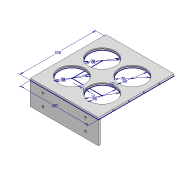
# Autodesk Inventor part: LensHolder
Saved by Autodesk Inventor 2020.3 (Build 243373010, 373A)
## iProperties
Created: 2020-12-03
Part Number: LensHolder
Material: Generic
Document SubType Name: Modeling
Designer: Yusuf
Mass: 169.587 g
Surface Area: 740.889 cm^2
Volume: 169.587 cm^3
Density: 1 g/cm^3
Appearance: Default
Author: Yusuf
Autodesk Inventor part; units mm, degrees
ref_plane "YZ Plane" through (0, 0, 0) normal (1, 0, 0) x (0, 1, 0)
ref_plane "XZ Plane" through (0, 0, 0) normal (0, 1, 0) x (-1, 0, 0)
ref_plane "XY Plane" through (0, 0, 0) normal (0, 0, 1) x (1, 0, 0)
sketch "Sketch1" plane through (0, 0, 0) normal (0, 1, 0) x (-1, 0, 0)
  line L0 (0, 0) -> (180, 0)
  line L1 (180, 0) -> (180, 200)
  line L2 (180, 200) -> (0, 200)
  line L3 (0, 200) -> (0, 0)
  circle A0 centre (130, 140) radius 35
  circle A1 centre (130, 60) radius 35
  circle A2 centre (50, 140) radius 35
  circle A3 centre (50, 60) radius 35
  line L4 (130, 140) -> (50, 140)
  line L5 (130, 140) -> (130, 60)
  circle A4 centre (130, 140) radius 34
  circle A5 centre (130, 60) radius 34
  circle A6 centre (50, 140) radius 34
  circle A7 centre (50, 60) radius 34
  point P0 (90, 140)
  point P1 (90, 200)
  point P2 (130, 100)
  point P3 (180, 100)
  dimension "d0" = 180
  dimension "d1" = 200
  dimension "d2" = 70
  dimension "d3" = 70
  dimension "d4" = 70
  dimension "d5" = 70
  dimension "d6" = 10
  dimension "d7" = 10
  dimension "d11" = 68
  dimension "d12" = 68
  dimension "d13" = 68
  dimension "d14" = 68
  constraints: 12 end point, 8 centre point, 4 coincident, 4 midpoint, 3 horizontal alignment, 3 vertical alignment, 2 horizontal, 2 parallel, 1 perpendicular, 1 vertical
  measures "d0" distance of L2.end L1.end
  measures "d1" distance of L1.end L0.end
  measures "d2" diameter of A0
  measures "d3" diameter of A1
  measures "d4" diameter of A2
  measures "d5" diameter of A3
  measures "d11" diameter of A4
  measures "d12" diameter of A5
  measures "d13" diameter of A6
  measures "d14" diameter of A7
extrude "Extrusion1" add sketch "Sketch1" along normal blind 5 contours L3 L2 L1 L0
extrude "Extrusion2" add sketch "Sketch1" along normal blind 3 contours A0 L5 A4 L4 | L4 A4 L5 A0 | A1 | A2 | A3
sketch "Sketch2" plane through (0, 0, 200) normal (1, 0, 0) x (0, 0, -1)
  circle A0 centre (40, 2.5) radius 1
  circle A1 centre (80, 2.5) radius 1
  circle A2 centre (120, 2.5) radius 1
  circle A3 centre (160, 2.5) radius 1
  line L0 (0, 0) -> (0, 5) projected
  line L1 (200, 0) -> (200, 5) projected
  line L2 (0, 5) -> (200, 5) projected
  dimension "d18" = 2
  dimension "d19" = 2
  dimension "d20" = 2
  dimension "d21" = 2
  dimension "d23" = 40
  dimension "d24" = 40
  dimension "d25" = 40
  dimension "d26" = 40
  dimension "d45" = 2.5
  constraints: 4 centre point, 3 horizontal alignment
  measures "d18" diameter of A0
  measures "d19" diameter of A1
  measures "d20" diameter of A2
  measures "d21" diameter of A3
  measures "d23" distance from line of L1 A3.centre
  measures "d24" distance of A3.centre A2.centre
  measures "d25" distance of A1.centre A2.centre
  measures "d26" distance of A1.centre A0.centre
  measures "d45" distance from line of L2 A1.centre
hole "Hole1" at (0, 2.5, 40) at (0, 2.5, 80) at (0, 2.5, 120) at (0, 2.5, 160) direction (-1, 0, 0) diameter 3.242 depth 11.8 thread size "M4x0.7" class "6H" standard "ANSI Metric M Profile"
sketch "Sketch3" plane through (0, 0, 0) normal (0, -1, 0) x (1, 0, 0)
  line L0 (0, 200) -> (0, 0) projected
  line L1 (-180, 0) -> (-180, 200) projected
  line L2 (0, 200) -> (-180, 200)
  line L3 (-180, 200) -> (-180, 194)
  line L4 (-180, 194) -> (0, 194)
  line L5 (0, 194) -> (0, 200)
  dimension "d35" = 6
  constraints: 8 end point, 2 parallel, 1 horizontal, 1 perpendicular, 1 point on line
  measures "d35" distance of L3.end L2.end
extrude "Extrusion3" add sketch "Sketch3" along normal blind 60
sketch "Sketch4" plane through (0, 0, 194) normal (0, 0, -1) x (-1, 0, 0)
  circle A0 centre (33.7554, -11.723) radius 5.5293
  circle A1 centre (33.7554, -43.277) radius 5.535
  circle A2 centre (146.2446, -11.723) radius 5.926
  circle A3 centre (146.2446, -43.277) radius 6.0534
  line L0 (33.7554, -11.723) -> (33.7554, -43.277)
  line L1 (33.7554, -11.723) -> (146.2446, -11.723)
  line L2 (0, 0) -> (180, 0) projected
  line L3 (0, -60) -> (0, 5) projected
  point P0 (90, -11.723)
  point P1 (90, 0)
  point P2 (33.7554, -27.5)
  point P3 (0, -27.5)
  constraints: 4 centre point, 4 end point, 4 midpoint, 3 horizontal alignment, 3 vertical alignment
hole "Hole2" at (-33.7554, -11.723, 194) at (-33.7554, -43.277, 194) at (-146.2446, -11.723, 194) at (-146.2446, -43.277, 194) direction (0, 0, 1) diameter 4.917 depth 17.1 thread size "M6x1" class "6H" standard "ANSI Metric M Profile"
body "Solid1"
